Autodesk Fusion 360 part; units mm, degrees
(part 4 of 5)
equation "d217 = SlotWidth"
equation "d218 = ( Depth ) - 2 * ( Wall + DeckClearance + RimBorder )"
equation "d219 = DeckThick"
equation "d221 = TouchChamfer"
equation "d222 = FootHeight"
equation "d224 = ( BaseX ) + ( 0 mm )"
equation "d225 = ( BaseY ) + ( 0 mm )"
equation "d226 = TowerWidth"
equation "d227 = Depth"
equation "d228 = PanHeight + RimLift"
equation "d232 = ( BaseX ) + ( Wall )"
equation "d234 = -( -( ( FootHeight ) + FloorMin + ( ( Depth ) - ( Wall ) ) * tan(DrainSlope) ) )"
equation "d235 = ( ( BaseY ) + ( Wall ) )"
equation "d236 = -( -( ( FootHeight ) + FloorMin + ( ( Depth ) - ( Depth ) ) * tan(DrainSlope) ) )"
equation "d237 = ( ( BaseY ) + ( Depth ) )"
equation "d238 = -( -( FootHeight + PanHeight + RimLift + 1 mm ) )"
equation "d239 = ( TowerWidth ) - 2 * Wall"
equation "d241 = FootHeight"
equation "d243 = ( ( BaseX ) + ( Wall ) )"
equation "d244 = ( ( BaseY ) + ( Wall ) )"
equation "d245 = ( ( BaseX ) + ( Wall + SeatReach ) )"
equation "d246 = ( ( BaseY ) + ( ( Wall ) + SeatLength / 2 ) )"
equation "d247 = ( ( BaseY ) + ( ( Wall ) + SeatLength ) )"
equation "d248 = PanHeight - DeckThick"
equation "d251 = SeatTipRadius"
equation "d252 = FootHeight"
equation "d254 = ( ( BaseX ) + ( Wall ) )"
equation "d255 = ( ( BaseY ) + ( ( Depth ) - Wall - SeatLength ) )"
equation "d256 = ( ( BaseX ) + ( Wall + SeatReach ) )"
equation "d257 = ( ( BaseY ) + ( ( ( Depth ) - Wall - SeatLength ) + SeatLength / 2 ) )"
equation "d258 = ( ( BaseY ) + ( ( ( Depth ) - Wall - SeatLength ) + SeatLength ) )"
equation "d259 = PanHeight - DeckThick"
equation "d262 = SeatTipRadius"
equation "d263 = FootHeight"
equation "d265 = ( ( BaseX ) + ( ( TowerWidth ) - Wall ) )"
equation "d266 = ( ( BaseY ) + ( Wall ) )"
equation "d267 = ( ( BaseX ) + ( ( TowerWidth ) - Wall - SeatReach ) )"
equation "d268 = ( ( BaseY ) + ( ( Wall ) + SeatLength / 2 ) )"
equation "d269 = ( ( BaseY ) + ( ( Wall ) + SeatLength ) )"
equation "d270 = PanHeight - DeckThick"
equation "d273 = SeatTipRadius"
equation "d274 = FootHeight"
equation "d276 = ( ( BaseX ) + ( ( TowerWidth ) - Wall ) )"
equation "d277 = ( ( BaseY ) + ( ( Depth ) - Wall - SeatLength ) )"
equation "d278 = ( ( BaseX ) + ( ( TowerWidth ) - Wall - SeatReach ) )"
equation "d279 = ( ( BaseY ) + ( ( ( Depth ) - Wall - SeatLength ) + SeatLength / 2 ) )"
equation "d280 = ( ( BaseY ) + ( ( ( Depth ) - Wall - SeatLength ) + SeatLength ) )"
equation "d281 = PanHeight - DeckThick"
equation "d284 = SeatTipRadius"
equation "d287 = ( BaseX ) + ( 3 mm )"
equation "d288 = ( BaseY ) + ( 0 mm )"
equation "d289 = RunnerWidth"
equation "d290 = ( Depth ) - 9 mm"
equation "d291 = FootHeight"
equation "d295 = ( BaseX ) + ( ( TowerWidth ) - 3 mm - RunnerWidth )"
equation "d296 = ( BaseY ) + ( 0 mm )"
equation "d297 = RunnerWidth"
equation "d298 = ( Depth ) - 9 mm"
equation "d299 = FootHeight"
equation "d301 = TouchChamfer"
equation "d302 = ( FootHeight ) + PanHeight - DeckThick"
equation "d304 = ( BaseX ) + ( Wall + DeckClearance )"
equation "d305 = ( BaseY ) + ( Wall + DeckClearance )"
equation "d306 = ( TowerWidth ) - 2 * ( Wall + DeckClearance )"
equation "d307 = ( Depth ) - 2 * ( Wall + DeckClearance )"
equation "d308 = DeckThick"
equation "d310 = ( FootHeight ) + PanHeight - DeckThick"
equation "d312 = ( BaseX ) + ( ( ( ( TowerWidth ) - ( 14 * SlotPitch + SlotWidth ) ) / 2 ) + ( 0 * SlotPitch ) )"
equation "d313 = ( BaseY ) + ( Wall + DeckClearance + RimBorder )"
equation "d314 = SlotWidth"
equation "d315 = ( Depth ) - 2 * ( Wall + DeckClearance + RimBorder )"
equation "d316 = DeckThick"
equation "d318 = ( FootHeight ) + PanHeight - DeckThick"
equation "d320 = ( BaseX ) + ( ( ( ( TowerWidth ) - ( 14 * SlotPitch + SlotWidth ) ) / 2 ) + ( 1 * SlotPitch ) )"
equation "d321 = ( BaseY ) + ( Wall + DeckClearance + RimBorder )"
equation "d322 = SlotWidth"
equation "d323 = ( Depth ) - 2 * ( Wall + DeckClearance + RimBorder )"
equation "d324 = DeckThick"
equation "d326 = ( FootHeight ) + PanHeight - DeckThick"
equation "d328 = ( BaseX ) + ( ( ( ( TowerWidth ) - ( 14 * SlotPitch + SlotWidth ) ) / 2 ) + ( 2 * SlotPitch ) )"
equation "d329 = ( BaseY ) + ( Wall + DeckClearance + RimBorder )"
equation "d330 = SlotWidth"
equation "d331 = ( Depth ) - 2 * ( Wall + DeckClearance + RimBorder )"
equation "d332 = DeckThick"
equation "d334 = ( FootHeight ) + PanHeight - DeckThick"
equation "d336 = ( BaseX ) + ( ( ( ( TowerWidth ) - ( 14 * SlotPitch + SlotWidth ) ) / 2 ) + ( 3 * SlotPitch ) )"
equation "d337 = ( BaseY ) + ( Wall + DeckClearance + RimBorder )"
equation "d338 = SlotWidth"
equation "d339 = ( Depth ) - 2 * ( Wall + DeckClearance + RimBorder )"
equation "d340 = DeckThick"
equation "d342 = ( FootHeight ) + PanHeight - DeckThick"
equation "d344 = ( BaseX ) + ( ( ( ( TowerWidth ) - ( 14 * SlotPitch + SlotWidth ) ) / 2 ) + ( 4 * SlotPitch ) )"
equation "d345 = ( BaseY ) + ( Wall + DeckClearance + RimBorder )"
equation "d346 = SlotWidth"
equation "d347 = ( Depth ) - 2 * ( Wall + DeckClearance + RimBorder )"
equation "d348 = DeckThick"
equation "d350 = ( FootHeight ) + PanHeight - DeckThick"
equation "d352 = ( BaseX ) + ( ( ( ( TowerWidth ) - ( 14 * SlotPitch + SlotWidth ) ) / 2 ) + ( 5 * SlotPitch ) )"
equation "d353 = ( BaseY ) + ( Wall + DeckClearance + RimBorder )"
equation "d354 = SlotWidth"
equation "d355 = ( Depth ) - 2 * ( Wall + DeckClearance + RimBorder )"
equation "d356 = DeckThick"
equation "d358 = ( FootHeight ) + PanHeight - DeckThick"
equation "d360 = ( BaseX ) + ( ( ( ( TowerWidth ) - ( 14 * SlotPitch + SlotWidth ) ) / 2 ) + ( 6 * SlotPitch ) )"
equation "d361 = ( BaseY ) + ( Wall + DeckClearance + RimBorder )"
equation "d362 = SlotWidth"
equation "d363 = ( Depth ) - 2 * ( Wall + DeckClearance + RimBorder )"
equation "d364 = DeckThick"
equation "d366 = ( FootHeight ) + PanHeight - DeckThick"
equation "d368 = ( BaseX ) + ( ( ( ( TowerWidth ) - ( 14 * SlotPitch + SlotWidth ) ) / 2 ) + ( 7 * SlotPitch ) )"
equation "d369 = ( BaseY ) + ( Wall + DeckClearance + RimBorder )"
equation "d370 = SlotWidth"
equation "d371 = ( Depth ) - 2 * ( Wall + DeckClearance + RimBorder )"
equation "d372 = DeckThick"
equation "d374 = ( FootHeight ) + PanHeight - DeckThick"
equation "d376 = ( BaseX ) + ( ( ( ( TowerWidth ) - ( 14 * SlotPitch + SlotWidth ) ) / 2 ) + ( 8 * SlotPitch ) )"
equation "d377 = ( BaseY ) + ( Wall + DeckClearance + RimBorder )"
equation "d378 = SlotWidth"
equation "d379 = ( Depth ) - 2 * ( Wall + DeckClearance + RimBorder )"
equation "d380 = DeckThick"
equation "d382 = ( FootHeight ) + PanHeight - DeckThick"
equation "d384 = ( BaseX ) + ( ( ( ( TowerWidth ) - ( 14 * SlotPitch + SlotWidth ) ) / 2 ) + ( 9 * SlotPitch ) )"
equation "d385 = ( BaseY ) + ( Wall + DeckClearance + RimBorder )"
equation "d386 = SlotWidth"
equation "d387 = ( Depth ) - 2 * ( Wall + DeckClearance + RimBorder )"
equation "d388 = DeckThick"
equation "d390 = ( FootHeight ) + PanHeight - DeckThick"
equation "d392 = ( BaseX ) + ( ( ( ( TowerWidth ) - ( 14 * SlotPitch + SlotWidth ) ) / 2 ) + ( 10 * SlotPitch ) )"
equation "d393 = ( BaseY ) + ( Wall + DeckClearance + RimBorder )"
equation "d394 = SlotWidth"
equation "d395 = ( Depth ) - 2 * ( Wall + DeckClearance + RimBorder )"
equation "d396 = DeckThick"
equation "d398 = ( FootHeight ) + PanHeight - DeckThick"
equation "d400 = ( BaseX ) + ( ( ( ( TowerWidth ) - ( 14 * SlotPitch + SlotWidth ) ) / 2 ) + ( 11 * SlotPitch ) )"
equation "d401 = ( BaseY ) + ( Wall + DeckClearance + RimBorder )"
equation "d402 = SlotWidth"
equation "d403 = ( Depth ) - 2 * ( Wall + DeckClearance + RimBorder )"
equation "d404 = DeckThick"
equation "d406 = ( FootHeight ) + PanHeight - DeckThick"
equation "d408 = ( BaseX ) + ( ( ( ( TowerWidth ) - ( 14 * SlotPitch + SlotWidth ) ) / 2 ) + ( 12 * SlotPitch ) )"
equation "d409 = ( BaseY ) + ( Wall + DeckClearance + RimBorder )"
equation "d410 = SlotWidth"
equation "d411 = ( Depth ) - 2 * ( Wall + DeckClearance + RimBorder )"
equation "d412 = DeckThick"
equation "d414 = ( FootHeight ) + PanHeight - DeckThick"
equation "d416 = ( BaseX ) + ( ( ( ( TowerWidth ) - ( 14 * SlotPitch + SlotWidth ) ) / 2 ) + ( 13 * SlotPitch ) )"
equation "d417 = ( BaseY ) + ( Wall + DeckClearance + RimBorder )"
equation "d418 = SlotWidth"
equation "d419 = ( Depth ) - 2 * ( Wall + DeckClearance + RimBorder )"
equation "d420 = DeckThick"
equation "d422 = ( FootHeight ) + PanHeight - DeckThick"
equation "d424 = ( BaseX ) + ( ( ( ( TowerWidth ) - ( 14 * SlotPitch + SlotWidth ) ) / 2 ) + ( 14 * SlotPitch ) )"
equation "d425 = ( BaseY ) + ( Wall + DeckClearance + RimBorder )"
equation "d426 = SlotWidth"
equation "d427 = ( Depth ) - 2 * ( Wall + DeckClearance + RimBorder )"
equation "d428 = DeckThick"
equation "d430 = TouchChamfer"
equation "d431 = FootHeight"
equation "d433 = ( BaseX + TowerWidth + ModuleGap ) + ( 0 mm )"
equation "d434 = ( BaseY ) + ( 0 mm )"
equation "d435 = LeftRun - TowerWidth - ModuleGap"
equation "d436 = Depth"
equation "d437 = PanHeight + RimLift"
equation "d441 = ( BaseX + TowerWidth + ModuleGap ) + ( Wall )"
equation "d443 = -( -( ( FootHeight ) + FloorMin + ( ( Depth ) - ( Wall ) ) * tan(DrainSlope) ) )"
equation "d444 = ( ( BaseY ) + ( Wall ) )"
equation "d445 = -( -( ( FootHeight ) + FloorMin + ( ( Depth ) - ( Depth ) ) * tan(DrainSlope) ) )"
equation "d446 = ( ( BaseY ) + ( Depth ) )"
equation "d447 = -( -( FootHeight + PanHeight + RimLift + 1 mm ) )"
equation "d448 = ( LeftRun - TowerWidth - ModuleGap ) - 2 * Wall"
equation "d450 = FootHeight"
equation "d452 = ( ( BaseX + TowerWidth + ModuleGap ) + ( Wall ) )"
equation "d453 = ( ( BaseY ) + ( Wall ) )"
equation "d454 = ( ( BaseX + TowerWidth + ModuleGap ) + ( Wall + SeatReach ) )"
equation "d455 = ( ( BaseY ) + ( ( Wall ) + SeatLength / 2 ) )"
equation "d456 = ( ( BaseY ) + ( ( Wall ) + SeatLength ) )"
equation "d457 = PanHeight - DeckThick"
equation "d460 = SeatTipRadius"
equation "d461 = FootHeight"
equation "d463 = ( ( BaseX + TowerWidth + ModuleGap ) + ( Wall ) )"
equation "d464 = ( ( BaseY ) + ( ( Depth ) - Wall - SeatLength ) )"
equation "d465 = ( ( BaseX + TowerWidth + ModuleGap ) + ( Wall + SeatReach ) )"
equation "d466 = ( ( BaseY ) + ( ( ( Depth ) - Wall - SeatLength ) + SeatLength / 2 ) )"
equation "d467 = ( ( BaseY ) + ( ( ( Depth ) - Wall - SeatLength ) + SeatLength ) )"
equation "d468 = PanHeight - DeckThick"
equation "d471 = SeatTipRadius"
equation "d472 = FootHeight"
equation "d474 = ( ( BaseX + TowerWidth + ModuleGap ) + ( ( LeftRun - TowerWidth - ModuleGap ) - Wall ) )"
equation "d475 = ( ( BaseY ) + ( Wall ) )"
equation "d476 = ( ( BaseX + TowerWidth + ModuleGap ) + ( ( LeftRun - TowerWidth - ModuleGap ) - Wall - SeatReach ) )"
equation "d477 = ( ( BaseY ) + ( ( Wall ) + SeatLength / 2 ) )"
equation "d478 = ( ( BaseY ) + ( ( Wall ) + SeatLength ) )"
equation "d479 = PanHeight - DeckThick"
equation "d482 = SeatTipRadius"
equation "d483 = FootHeight"
equation "d485 = ( ( BaseX + TowerWidth + ModuleGap ) + ( ( LeftRun - TowerWidth - ModuleGap ) - Wall ) )"
equation "d486 = ( ( BaseY ) + ( ( Depth ) - Wall - SeatLength ) )"
equation "d487 = ( ( BaseX + TowerWidth + ModuleGap ) + ( ( LeftRun - TowerWidth - ModuleGap ) - Wall - SeatReach ) )"
equation "d488 = ( ( BaseY ) + ( ( ( Depth ) - Wall - SeatLength ) + SeatLength / 2 ) )"
equation "d489 = ( ( BaseY ) + ( ( ( Depth ) - Wall - SeatLength ) + SeatLength ) )"
equation "d490 = PanHeight - DeckThick"
equation "d493 = SeatTipRadius"
equation "d496 = ( BaseX + TowerWidth + ModuleGap ) + ( 3 mm )"
equation "d497 = ( BaseY ) + ( 0 mm )"
equation "d498 = RunnerWidth"
equation "d499 = ( Depth ) - 9 mm"
equation "d500 = FootHeight"
equation "d504 = ( BaseX + TowerWidth + ModuleGap ) + ( ( LeftRun - TowerWidth - ModuleGap ) - 3 mm - RunnerWidth )"
equation "d505 = ( BaseY ) + ( 0 mm )"
equation "d506 = RunnerWidth"
equation "d507 = ( Depth ) - 9 mm"
equation "d508 = FootHeight"
equation "d510 = TouchChamfer"
equation "d511 = ( FootHeight ) + PanHeight - DeckThick"
equation "d513 = ( BaseX + TowerWidth + ModuleGap ) + ( Wall + DeckClearance )"
equation "d514 = ( BaseY ) + ( Wall + DeckClearance )"
equation "d515 = ( LeftRun - TowerWidth - ModuleGap ) - 2 * ( Wall + DeckClearance )"
equation "d516 = ( Depth ) - 2 * ( Wall + DeckClearance )"
equation "d517 = DeckThick"
equation "d519 = ( FootHeight ) + PanHeight - DeckThick"
equation "d521 = ( BaseX + TowerWidth + ModuleGap ) + ( ( ( ( LeftRun - TowerWidth - ModuleGap ) - ( 16 * SlotPitch + SlotWidth ) ) / 2 ) + ( 0 * SlotPitch ) )"
equation "d522 = ( BaseY ) + ( Wall + DeckClearance + RimBorder )"
equation "d523 = SlotWidth"
equation "d524 = ( Depth ) - 2 * ( Wall + DeckClearance + RimBorder )"
equation "d525 = DeckThick"
equation "d527 = ( FootHeight ) + PanHeight - DeckThick"
equation "d529 = ( BaseX + TowerWidth + ModuleGap ) + ( ( ( ( LeftRun - TowerWidth - ModuleGap ) - ( 16 * SlotPitch + SlotWidth ) ) / 2 ) + ( 1 * SlotPitch ) )"
equation "d530 = ( BaseY ) + ( Wall + DeckClearance + RimBorder )"
equation "d531 = SlotWidth"
equation "d532 = ( Depth ) - 2 * ( Wall + DeckClearance + RimBorder )"
equation "d533 = DeckThick"
equation "d535 = ( FootHeight ) + PanHeight - DeckThick"
equation "d537 = ( BaseX + TowerWidth + ModuleGap ) + ( ( ( ( LeftRun - TowerWidth - ModuleGap ) - ( 16 * SlotPitch + SlotWidth ) ) / 2 ) + ( 2 * SlotPitch ) )"
equation "d538 = ( BaseY ) + ( Wall + DeckClearance + RimBorder )"
equation "d539 = SlotWidth"
equation "d540 = ( Depth ) - 2 * ( Wall + DeckClearance + RimBorder )"
equation "d541 = DeckThick"
equation "d543 = ( FootHeight ) + PanHeight - DeckThick"
equation "d545 = ( BaseX + TowerWidth + ModuleGap ) + ( ( ( ( LeftRun - TowerWidth - ModuleGap ) - ( 16 * SlotPitch + SlotWidth ) ) / 2 ) + ( 3 * SlotPitch ) )"
equation "d546 = ( BaseY ) + ( Wall + DeckClearance + RimBorder )"
equation "d547 = SlotWidth"
equation "d548 = ( Depth ) - 2 * ( Wall + DeckClearance + RimBorder )"
equation "d549 = DeckThick"
equation "d551 = ( FootHeight ) + PanHeight - DeckThick"
equation "d553 = ( BaseX + TowerWidth + ModuleGap ) + ( ( ( ( LeftRun - TowerWidth - ModuleGap ) - ( 16 * SlotPitch + SlotWidth ) ) / 2 ) + ( 4 * SlotPitch ) )"
equation "d554 = ( BaseY ) + ( Wall + DeckClearance + RimBorder )"
equation "d555 = SlotWidth"
equation "d556 = ( Depth ) - 2 * ( Wall + DeckClearance + RimBorder )"
equation "d557 = DeckThick"
equation "d559 = ( FootHeight ) + PanHeight - DeckThick"
equation "d561 = ( BaseX + TowerWidth + ModuleGap ) + ( ( ( ( LeftRun - TowerWidth - ModuleGap ) - ( 16 * SlotPitch + SlotWidth ) ) / 2 ) + ( 5 * SlotPitch ) )"
equation "d562 = ( BaseY ) + ( Wall + DeckClearance + RimBorder )"
equation "d563 = SlotWidth"
equation "d564 = ( Depth ) - 2 * ( Wall + DeckClearance + RimBorder )"
equation "d565 = DeckThick"
equation "d567 = ( FootHeight ) + PanHeight - DeckThick"
equation "d569 = ( BaseX + TowerWidth + ModuleGap ) + ( ( ( ( LeftRun - TowerWidth - ModuleGap ) - ( 16 * SlotPitch + SlotWidth ) ) / 2 ) + ( 6 * SlotPitch ) )"
equation "d570 = ( BaseY ) + ( Wall + DeckClearance + RimBorder )"
equation "d571 = SlotWidth"
equation "d572 = ( Depth ) - 2 * ( Wall + DeckClearance + RimBorder )"
equation "d573 = DeckThick"
equation "d575 = ( FootHeight ) + PanHeight - DeckThick"
equation "d577 = ( BaseX + TowerWidth + ModuleGap ) + ( ( ( ( LeftRun - TowerWidth - ModuleGap ) - ( 16 * SlotPitch + SlotWidth ) ) / 2 ) + ( 7 * SlotPitch ) )"
equation "d578 = ( BaseY ) + ( Wall + DeckClearance + RimBorder )"
equation "d579 = SlotWidth"
equation "d580 = ( Depth ) - 2 * ( Wall + DeckClearance + RimBorder )"
equation "d581 = DeckThick"
equation "d583 = ( FootHeight ) + PanHeight - DeckThick"
equation "d585 = ( BaseX + TowerWidth + ModuleGap ) + ( ( ( ( LeftRun - TowerWidth - ModuleGap ) - ( 16 * SlotPitch + SlotWidth ) ) / 2 ) + ( 8 * SlotPitch ) )"
equation "d586 = ( BaseY ) + ( Wall + DeckClearance + RimBorder )"
equation "d587 = SlotWidth"
equation "d588 = ( Depth ) - 2 * ( Wall + DeckClearance + RimBorder )"
equation "d589 = DeckThick"
equation "d591 = ( FootHeight ) + PanHeight - DeckThick"
equation "d593 = ( BaseX + TowerWidth + ModuleGap ) + ( ( ( ( LeftRun - TowerWidth - ModuleGap ) - ( 16 * SlotPitch + SlotWidth ) ) / 2 ) + ( 9 * SlotPitch ) )"
equation "d594 = ( BaseY ) + ( Wall + DeckClearance + RimBorder )"
equation "d595 = SlotWidth"
equation "d596 = ( Depth ) - 2 * ( Wall + DeckClearance + RimBorder )"
equation "d597 = DeckThick"
equation "d599 = ( FootHeight ) + PanHeight - DeckThick"
equation "d601 = ( BaseX + TowerWidth + ModuleGap ) + ( ( ( ( LeftRun - TowerWidth - ModuleGap ) - ( 16 * SlotPitch + SlotWidth ) ) / 2 ) + ( 10 * SlotPitch ) )"
equation "d602 = ( BaseY ) + ( Wall + DeckClearance + RimBorder )"
equation "d603 = SlotWidth"
equation "d604 = ( Depth ) - 2 * ( Wall + DeckClearance + RimBorder )"
equation "d605 = DeckThick"
equation "d607 = ( FootHeight ) + PanHeight - DeckThick"
equation "d609 = ( BaseX + TowerWidth + ModuleGap ) + ( ( ( ( LeftRun - TowerWidth - ModuleGap ) - ( 16 * SlotPitch + SlotWidth ) ) / 2 ) + ( 11 * SlotPitch ) )"
equation "d610 = ( BaseY ) + ( Wall + DeckClearance + RimBorder )"
equation "d611 = SlotWidth"
equation "d612 = ( Depth ) - 2 * ( Wall + DeckClearance + RimBorder )"
equation "d613 = DeckThick"
equation "d615 = ( FootHeight ) + PanHeight - DeckThick"
equation "d617 = ( BaseX + TowerWidth + ModuleGap ) + ( ( ( ( LeftRun - TowerWidth - ModuleGap ) - ( 16 * SlotPitch + SlotWidth ) ) / 2 ) + ( 12 * SlotPitch ) )"
equation "d618 = ( BaseY ) + ( Wall + DeckClearance + RimBorder )"
equation "d619 = SlotWidth"
equation "d620 = ( Depth ) - 2 * ( Wall + DeckClearance + RimBorder )"
equation "d621 = DeckThick"
equation "d623 = ( FootHeight ) + PanHeight - DeckThick"
equation "d625 = ( BaseX + TowerWidth + ModuleGap ) + ( ( ( ( LeftRun - TowerWidth - ModuleGap ) - ( 16 * SlotPitch + SlotWidth ) ) / 2 ) + ( 13 * SlotPitch ) )"
equation "d626 = ( BaseY ) + ( Wall + DeckClearance + RimBorder )"
equation "d627 = SlotWidth"
equation "d628 = ( Depth ) - 2 * ( Wall + DeckClearance + RimBorder )"
equation "d629 = DeckThick"
equation "d631 = ( FootHeight ) + PanHeight - DeckThick"
equation "d633 = ( BaseX + TowerWidth + ModuleGap ) + ( ( ( ( LeftRun - TowerWidth - ModuleGap ) - ( 16 * SlotPitch + SlotWidth ) ) / 2 ) + ( 14 * SlotPitch ) )"
equation "d634 = ( BaseY ) + ( Wall + DeckClearance + RimBorder )"
equation "d635 = SlotWidth"
equation "d636 = ( Depth ) - 2 * ( Wall + DeckClearance + RimBorder )"
equation "d637 = DeckThick"
equation "d639 = ( FootHeight ) + PanHeight - DeckThick"
equation "d641 = ( BaseX + TowerWidth + ModuleGap ) + ( ( ( ( LeftRun - TowerWidth - ModuleGap ) - ( 16 * SlotPitch + SlotWidth ) ) / 2 ) + ( 15 * SlotPitch ) )"
equation "d642 = ( BaseY ) + ( Wall + DeckClearance + RimBorder )"
equation "d643 = SlotWidth"
equation "d644 = ( Depth ) - 2 * ( Wall + DeckClearance + RimBorder )"
equation "d645 = DeckThick"
equation "d647 = ( FootHeight ) + PanHeight - DeckThick"
equation "d649 = ( BaseX + TowerWidth + ModuleGap ) + ( ( ( ( LeftRun - TowerWidth - ModuleGap ) - ( 16 * SlotPitch + SlotWidth ) ) / 2 ) + ( 16 * SlotPitch ) )"
equation "d650 = ( BaseY ) + ( Wall + DeckClearance + RimBorder )"
equation "d651 = SlotWidth"
equation "d652 = ( Depth ) - 2 * ( Wall + DeckClearance + RimBorder )"
equation "d653 = DeckThick"
equation "d655 = TouchChamfer"
equation "d656 = FootHeight"
equation "d658 = ( BaseX + LeftRun + FaucetGap + ( RightRun + ModuleGap ) / 2 ) + ( 0 mm )"
equation "d659 = ( BaseY ) + ( 0 mm )"
equation "d660 = ( RightRun - ModuleGap ) / 2"
equation "d661 = Depth"
equation "d662 = PanHeight + RimLift"
equation "d666 = ( BaseX + LeftRun + FaucetGap + ( RightRun + ModuleGap ) / 2 ) + ( Wall )"
equation "d668 = -( -( ( FootHeight ) + FloorMin + ( ( Depth ) - ( Wall ) ) * tan(DrainSlope) ) )"
equation "d669 = ( ( BaseY ) + ( Wall ) )"
equation "d670 = -( -( ( FootHeight ) + FloorMin + ( ( Depth ) - ( Depth ) ) * tan(DrainSlope) ) )"
equation "d671 = ( ( BaseY ) + ( Depth ) )"
equation "d672 = -( -( FootHeight + PanHeight + RimLift + 1 mm ) )"
equation "d673 = ( ( RightRun - ModuleGap ) / 2 ) - 2 * Wall"
equation "d675 = FootHeight"
equation "d677 = ( ( BaseX + LeftRun + FaucetGap + ( RightRun + ModuleGap ) / 2 ) + ( Wall ) )"
equation "d678 = ( ( BaseY ) + ( Wall ) )"
equation "d679 = ( ( BaseX + LeftRun + FaucetGap + ( RightRun + ModuleGap ) / 2 ) + ( Wall + SeatReach ) )"
equation "d680 = ( ( BaseY ) + ( ( Wall ) + SeatLength / 2 ) )"
equation "d681 = ( ( BaseY ) + ( ( Wall ) + SeatLength ) )"
equation "d682 = PanHeight - DeckThick"
equation "d685 = SeatTipRadius"
equation "d686 = FootHeight"
equation "d688 = ( ( BaseX + LeftRun + FaucetGap + ( RightRun + ModuleGap ) / 2 ) + ( Wall ) )"
equation "d689 = ( ( BaseY ) + ( ( Depth ) - Wall - SeatLength ) )"
equation "d690 = ( ( BaseX + LeftRun + FaucetGap + ( RightRun + ModuleGap ) / 2 ) + ( Wall + SeatReach ) )"
equation "d691 = ( ( BaseY ) + ( ( ( Depth ) - Wall - SeatLength ) + SeatLength / 2 ) )"
equation "d692 = ( ( BaseY ) + ( ( ( Depth ) - Wall - SeatLength ) + SeatLength ) )"
equation "d693 = PanHeight - DeckThick"
equation "d696 = SeatTipRadius"
equation "d697 = FootHeight"
equation "d699 = ( ( BaseX + LeftRun + FaucetGap + ( RightRun + ModuleGap ) / 2 ) + ( ( ( RightRun - ModuleGap ) / 2 ) - Wall ) )"
equation "d700 = ( ( BaseY ) + ( Wall ) )"
equation "d701 = ( ( BaseX + LeftRun + FaucetGap + ( RightRun + ModuleGap ) / 2 ) + ( ( ( RightRun - ModuleGap ) / 2 ) - Wall - SeatReach ) )"
equation "d702 = ( ( BaseY ) + ( ( Wall ) + SeatLength / 2 ) )"
equation "d703 = ( ( BaseY ) + ( ( Wall ) + SeatLength ) )"
equation "d704 = PanHeight - DeckThick"
equation "d707 = SeatTipRadius"
equation "d708 = FootHeight"
equation "d710 = ( ( BaseX + LeftRun + FaucetGap + ( RightRun + ModuleGap ) / 2 ) + ( ( ( RightRun - ModuleGap ) / 2 ) - Wall ) )"
equation "d711 = ( ( BaseY ) + ( ( Depth ) - Wall - SeatLength ) )"
equation "d712 = ( ( BaseX + LeftRun + FaucetGap + ( RightRun + ModuleGap ) / 2 ) + ( ( ( RightRun - ModuleGap ) / 2 ) - Wall - SeatReach ) )"
equation "d713 = ( ( BaseY ) + ( ( ( Depth ) - Wall - SeatLength ) + SeatLength / 2 ) )"
equation "d714 = ( ( BaseY ) + ( ( ( Depth ) - Wall - SeatLength ) + SeatLength ) )"
equation "d715 = PanHeight - DeckThick"
equation "d718 = SeatTipRadius"
equation "d721 = ( BaseX + LeftRun + FaucetGap + ( RightRun + ModuleGap ) / 2 ) + ( 3 mm )"
equation "d722 = ( BaseY ) + ( 0 mm )"
equation "d723 = RunnerWidth"
equation "d724 = ( Depth ) - 9 mm"
equation "d725 = FootHeight"
equation "d729 = ( BaseX + LeftRun + FaucetGap + ( RightRun + ModuleGap ) / 2 ) + ( ( ( RightRun - ModuleGap ) / 2 ) - 3 mm - RunnerWidth )"
equation "d730 = ( BaseY ) + ( 0 mm )"
equation "d731 = RunnerWidth"
equation "d732 = ( Depth ) - 9 mm"
equation "d733 = FootHeight"
equation "d735 = TouchChamfer"
equation "d736 = ( FootHeight ) + PanHeight - DeckThick"
equation "d738 = ( BaseX + LeftRun + FaucetGap + ( RightRun + ModuleGap ) / 2 ) + ( Wall + DeckClearance )"
equation "d739 = ( BaseY ) + ( Wall + DeckClearance )"
equation "d740 = ( ( RightRun - ModuleGap ) / 2 ) - 2 * ( Wall + DeckClearance )"
equation "d741 = ( Depth ) - 2 * ( Wall + DeckClearance )"
equation "d742 = DeckThick"
equation "d744 = ( FootHeight ) + PanHeight - DeckThick"
equation "d746 = ( BaseX + LeftRun + FaucetGap + ( RightRun + ModuleGap ) / 2 ) + ( ( ( ( ( RightRun - ModuleGap ) / 2 ) - ( 10 * SlotPitch + SlotWidth ) ) / 2 ) + ( 0 * SlotPitch ) )"
equation "d747 = ( BaseY ) + ( Wall + DeckClearance + RimBorder )"
equation "d748 = SlotWidth"
equation "d749 = ( Depth ) - 2 * ( Wall + DeckClearance + RimBorder )"
equation "d750 = DeckThick"
equation "d752 = ( FootHeight ) + PanHeight - DeckThick"
equation "d754 = ( BaseX + LeftRun + FaucetGap + ( RightRun + ModuleGap ) / 2 ) + ( ( ( ( ( RightRun - ModuleGap ) / 2 ) - ( 10 * SlotPitch + SlotWidth ) ) / 2 ) + ( 1 * SlotPitch ) )"
equation "d755 = ( BaseY ) + ( Wall + DeckClearance + RimBorder )"
equation "d756 = SlotWidth"
equation "d757 = ( Depth ) - 2 * ( Wall + DeckClearance + RimBorder )"
equation "d758 = DeckThick"
equation "d760 = ( FootHeight ) + PanHeight - DeckThick"
equation "d762 = ( BaseX + LeftRun + FaucetGap + ( RightRun + ModuleGap ) / 2 ) + ( ( ( ( ( RightRun - ModuleGap ) / 2 ) - ( 10 * SlotPitch + SlotWidth ) ) / 2 ) + ( 2 * SlotPitch ) )"
equation "d763 = ( BaseY ) + ( Wall + DeckClearance + RimBorder )"
equation "d764 = SlotWidth"
equation "d765 = ( Depth ) - 2 * ( Wall + DeckClearance + RimBorder )"
equation "d766 = DeckThick"
equation "d768 = ( FootHeight ) + PanHeight - DeckThick"
equation "d770 = ( BaseX + LeftRun + FaucetGap + ( RightRun + ModuleGap ) / 2 ) + ( ( ( ( ( RightRun - ModuleGap ) / 2 ) - ( 10 * SlotPitch + SlotWidth ) ) / 2 ) + ( 3 * SlotPitch ) )"
equation "d771 = ( BaseY ) + ( Wall + DeckClearance + RimBorder )"
equation "d772 = SlotWidth"
equation "d773 = ( Depth ) - 2 * ( Wall + DeckClearance + RimBorder )"
equation "d774 = DeckThick"
equation "d776 = ( FootHeight ) + PanHeight - DeckThick"
equation "d778 = ( BaseX + LeftRun + FaucetGap + ( RightRun + ModuleGap ) / 2 ) + ( ( ( ( ( RightRun - ModuleGap ) / 2 ) - ( 10 * SlotPitch + SlotWidth ) ) / 2 ) + ( 4 * SlotPitch ) )"
equation "d779 = ( BaseY ) + ( Wall + DeckClearance + RimBorder )"
equation "d780 = SlotWidth"
equation "d781 = ( Depth ) - 2 * ( Wall + DeckClearance + RimBorder )"
equation "d782 = DeckThick"
equation "d784 = ( FootHeight ) + PanHeight - DeckThick"
equation "d786 = ( BaseX + LeftRun + FaucetGap + ( RightRun + ModuleGap ) / 2 ) + ( ( ( ( ( RightRun - ModuleGap ) / 2 ) - ( 10 * SlotPitch + SlotWidth ) ) / 2 ) + ( 5 * SlotPitch ) )"
equation "d787 = ( BaseY ) + ( Wall + DeckClearance + RimBorder )"
equation "d788 = SlotWidth"
equation "d789 = ( Depth ) - 2 * ( Wall + DeckClearance + RimBorder )"
equation "d790 = DeckThick"
equation "d792 = ( FootHeight ) + PanHeight - DeckThick"
equation "d794 = ( BaseX + LeftRun + FaucetGap + ( RightRun + ModuleGap ) / 2 ) + ( ( ( ( ( RightRun - ModuleGap ) / 2 ) - ( 10 * SlotPitch + SlotWidth ) ) / 2 ) + ( 6 * SlotPitch ) )"
equation "d795 = ( BaseY ) + ( Wall + DeckClearance + RimBorder )"
equation "d796 = SlotWidth"
equation "d797 = ( Depth ) - 2 * ( Wall + DeckClearance + RimBorder )"
equation "d798 = DeckThick"
equation "d800 = ( FootHeight ) + PanHeight - DeckThick"
equation "d802 = ( BaseX + LeftRun + FaucetGap + ( RightRun + ModuleGap ) / 2 ) + ( ( ( ( ( RightRun - ModuleGap ) / 2 ) - ( 10 * SlotPitch + SlotWidth ) ) / 2 ) + ( 7 * SlotPitch ) )"
equation "d803 = ( BaseY ) + ( Wall + DeckClearance + RimBorder )"
equation "d804 = SlotWidth"
equation "d805 = ( Depth ) - 2 * ( Wall + DeckClearance + RimBorder )"
equation "d806 = DeckThick"
equation "d808 = ( FootHeight ) + PanHeight - DeckThick"
equation "d810 = ( BaseX + LeftRun + FaucetGap + ( RightRun + ModuleGap ) / 2 ) + ( ( ( ( ( RightRun - ModuleGap ) / 2 ) - ( 10 * SlotPitch + SlotWidth ) ) / 2 ) + ( 8 * SlotPitch ) )"
equation "d811 = ( BaseY ) + ( Wall + DeckClearance + RimBorder )"
equation "d812 = SlotWidth"
equation "d813 = ( Depth ) - 2 * ( Wall + DeckClearance + RimBorder )"
equation "d814 = DeckThick"
equation "d816 = ( FootHeight ) + PanHeight - DeckThick"
equation "d818 = ( BaseX + LeftRun + FaucetGap + ( RightRun + ModuleGap ) / 2 ) + ( ( ( ( ( RightRun - ModuleGap ) / 2 ) - ( 10 * SlotPitch + SlotWidth ) ) / 2 ) + ( 9 * SlotPitch ) )"
equation "d819 = ( BaseY ) + ( Wall + DeckClearance + RimBorder )"
equation "d820 = SlotWidth"
equation "d821 = ( Depth ) - 2 * ( Wall + DeckClearance + RimBorder )"
equation "d822 = DeckThick"
equation "d824 = ( FootHeight ) + PanHeight - DeckThick"
equation "d826 = ( BaseX + LeftRun + FaucetGap + ( RightRun + ModuleGap ) / 2 ) + ( ( ( ( ( RightRun - ModuleGap ) / 2 ) - ( 10 * SlotPitch + SlotWidth ) ) / 2 ) + ( 10 * SlotPitch ) )"
equation "d827 = ( BaseY ) + ( Wall + DeckClearance + RimBorder )"
equation "d828 = SlotWidth"
equation "d829 = ( Depth ) - 2 * ( Wall + DeckClearance + RimBorder )"
equation "d830 = DeckThick"
equation "d832 = TouchChamfer"
equation "d833 = FootHeight"
equation "d835 = ( BaseX ) + ( 0 mm )"
equation "d836 = ( BaseY + Depth + ModuleGap ) + ( ( LeftReach ) - ( ( 0 mm ) + ( LeftReach ) ) )"
equation "d837 = LeftSideDepth"
equation "d838 = LeftReach"
equation "d839 = PanHeight + RimLift"
equation "d843 = ( BaseY + Depth + ModuleGap ) + ( ( LeftReach ) - ( Wall ) )"
equation "d845 = ( ( BaseX ) + ( Wall ) )"
equation "d846 = -( -( ( FootHeight ) + FloorMin + ( ( LeftSideDepth ) - ( Wall ) ) * tan(DrainSlope) ) )"
equation "d847 = ( ( BaseX ) + ( LeftSideDepth ) )"
equation "d848 = -( -( ( FootHeight ) + FloorMin + ( ( LeftSideDepth ) - ( LeftSideDepth ) ) * tan(DrainSlope) ) )"
equation "d849 = -( -( FootHeight + PanHeight + RimLift + 1 mm ) )"
equation "d850 = -( -( -( ( LeftReach ) - 2 * Wall ) ) )"
equation "d852 = FootHeight"
equation "d854 = ( ( BaseX ) + ( Wall ) )"
equation "d855 = ( ( BaseY + Depth + ModuleGap ) + ( ( LeftReach ) - ( Wall ) ) )"
equation "d856 = ( ( BaseX ) + ( ( Wall ) + SeatLength / 2 ) )"
equation "d857 = ( ( BaseY + Depth + ModuleGap ) + ( ( LeftReach ) - ( Wall + SeatReach ) ) )"
equation "d858 = ( ( BaseX ) + ( ( Wall ) + SeatLength ) )"
equation "d859 = PanHeight - DeckThick"
equation "d862 = SeatTipRadius"
equation "d863 = FootHeight"
equation "d865 = ( ( BaseX ) + ( ( LeftSideDepth ) - Wall - SeatLength ) )"
equation "d866 = ( ( BaseY + Depth + ModuleGap ) + ( ( LeftReach ) - ( Wall ) ) )"
equation "d867 = ( ( BaseX ) + ( ( ( LeftSideDepth ) - Wall - SeatLength ) + SeatLength / 2 ) )"
equation "d868 = ( ( BaseY + Depth + ModuleGap ) + ( ( LeftReach ) - ( Wall + SeatReach ) ) )"
equation "d869 = ( ( BaseX ) + ( ( ( LeftSideDepth ) - Wall - SeatLength ) + SeatLength ) )"
equation "d870 = PanHeight - DeckThick"
equation "d873 = SeatTipRadius"
equation "d874 = FootHeight"
equation "d876 = ( ( BaseX ) + ( Wall ) )"
equation "d877 = ( ( BaseY + Depth + ModuleGap ) + ( ( LeftReach ) - ( ( LeftReach ) - Wall ) ) )"
equation "d878 = ( ( BaseX ) + ( ( Wall ) + SeatLength / 2 ) )"
equation "d879 = ( ( BaseY + Depth + ModuleGap ) + ( ( LeftReach ) - ( ( LeftReach ) - Wall - SeatReach ) ) )"
equation "d880 = ( ( BaseX ) + ( ( Wall ) + SeatLength ) )"
equation "d881 = PanHeight - DeckThick"
equation "d884 = SeatTipRadius"
equation "d885 = FootHeight"
equation "d887 = ( ( BaseX ) + ( ( LeftSideDepth ) - Wall - SeatLength ) )"
equation "d888 = ( ( BaseY + Depth + ModuleGap ) + ( ( LeftReach ) - ( ( LeftReach ) - Wall ) ) )"
equation "d889 = ( ( BaseX ) + ( ( ( LeftSideDepth ) - Wall - SeatLength ) + SeatLength / 2 ) )"
equation "d890 = ( ( BaseY + Depth + ModuleGap ) + ( ( LeftReach ) - ( ( LeftReach ) - Wall - SeatReach ) ) )"
equation "d891 = ( ( BaseX ) + ( ( ( LeftSideDepth ) - Wall - SeatLength ) + SeatLength ) )"
equation "d892 = PanHeight - DeckThick"
equation "d895 = SeatTipRadius"
equation "d898 = ( BaseX ) + ( 0 mm )"
equation "d899 = ( BaseY + Depth + ModuleGap ) + ( ( LeftReach ) - ( ( 3 mm ) + ( RunnerWidth ) ) )"
equation "d900 = ( LeftSideDepth ) - 9 mm"
equation "d901 = RunnerWidth"
equation "d902 = FootHeight"
equation "d906 = ( BaseX ) + ( 0 mm )"
equation "d907 = ( BaseY + Depth + ModuleGap ) + ( ( LeftReach ) - ( ( ( LeftReach ) - 3 mm - RunnerWidth ) + ( RunnerWidth ) ) )"
equation "d908 = ( LeftSideDepth ) - 9 mm"
equation "d909 = RunnerWidth"
equation "d910 = FootHeight"
equation "d912 = TouchChamfer"
equation "d913 = ( FootHeight ) + PanHeight - DeckThick"
equation "d915 = ( BaseX ) + ( Wall + DeckClearance )"
equation "d916 = ( BaseY + Depth + ModuleGap ) + ( ( LeftReach ) - ( ( Wall + DeckClearance ) + ( ( LeftReach ) - 2 * ( Wall + DeckClearance ) ) ) )"
equation "d917 = ( LeftSideDepth ) - 2 * ( Wall + DeckClearance )"
equation "d918 = ( LeftReach ) - 2 * ( Wall + DeckClearance )"
equation "d919 = DeckThick"
equation "d921 = ( FootHeight ) + PanHeight - DeckThick"
equation "d923 = ( BaseX ) + ( Wall + DeckClearance + RimBorder )"
equation "d924 = ( BaseY + Depth + ModuleGap ) + ( ( LeftReach ) - ( ( ( ( ( LeftReach ) - ( 14 * SlotPitch + SlotWidth ) ) / 2 ) + ( 0 * SlotPitch ) ) + ( SlotWidth ) ) )"
equation "d925 = ( LeftSideDepth ) - 2 * ( Wall + DeckClearance + RimBorder )"
equation "d926 = SlotWidth"
equation "d927 = DeckThick"
equation "d929 = ( FootHeight ) + PanHeight - DeckThick"
equation "d931 = ( BaseX ) + ( Wall + DeckClearance + RimBorder )"
equation "d932 = ( BaseY + Depth + ModuleGap ) + ( ( LeftReach ) - ( ( ( ( ( LeftReach ) - ( 14 * SlotPitch + SlotWidth ) ) / 2 ) + ( 1 * SlotPitch ) ) + ( SlotWidth ) ) )"
equation "d933 = ( LeftSideDepth ) - 2 * ( Wall + DeckClearance + RimBorder )"
equation "d934 = SlotWidth"
equation "d935 = DeckThick"
equation "d937 = ( FootHeight ) + PanHeight - DeckThick"
equation "d939 = ( BaseX ) + ( Wall + DeckClearance + RimBorder )"
equation "d940 = ( BaseY + Depth + ModuleGap ) + ( ( LeftReach ) - ( ( ( ( ( LeftReach ) - ( 14 * SlotPitch + SlotWidth ) ) / 2 ) + ( 2 * SlotPitch ) ) + ( SlotWidth ) ) )"
equation "d941 = ( LeftSideDepth ) - 2 * ( Wall + DeckClearance + RimBorder )"
equation "d942 = SlotWidth"
equation "d943 = DeckThick"
equation "d945 = ( FootHeight ) + PanHeight - DeckThick"
equation "d947 = ( BaseX ) + ( Wall + DeckClearance + RimBorder )"
equation "d948 = ( BaseY + Depth + ModuleGap ) + ( ( LeftReach ) - ( ( ( ( ( LeftReach ) - ( 14 * SlotPitch + SlotWidth ) ) / 2 ) + ( 3 * SlotPitch ) ) + ( SlotWidth ) ) )"
equation "d949 = ( LeftSideDepth ) - 2 * ( Wall + DeckClearance + RimBorder )"
equation "d950 = SlotWidth"
equation "d951 = DeckThick"
equation "d953 = ( FootHeight ) + PanHeight - DeckThick"
equation "d955 = ( BaseX ) + ( Wall + DeckClearance + RimBorder )"
equation "d956 = ( BaseY + Depth + ModuleGap ) + ( ( LeftReach ) - ( ( ( ( ( LeftReach ) - ( 14 * SlotPitch + SlotWidth ) ) / 2 ) + ( 4 * SlotPitch ) ) + ( SlotWidth ) ) )"
equation "d957 = ( LeftSideDepth ) - 2 * ( Wall + DeckClearance + RimBorder )"
equation "d958 = SlotWidth"
equation "d959 = DeckThick"
equation "d961 = ( FootHeight ) + PanHeight - DeckThick"
equation "d963 = ( BaseX ) + ( Wall + DeckClearance + RimBorder )"
equation "d964 = ( BaseY + Depth + ModuleGap ) + ( ( LeftReach ) - ( ( ( ( ( LeftReach ) - ( 14 * SlotPitch + SlotWidth ) ) / 2 ) + ( 5 * SlotPitch ) ) + ( SlotWidth ) ) )"
equation "d965 = ( LeftSideDepth ) - 2 * ( Wall + DeckClearance + RimBorder )"
equation "d966 = SlotWidth"
equation "d967 = DeckThick"
equation "d969 = ( FootHeight ) + PanHeight - DeckThick"
equation "d971 = ( BaseX ) + ( Wall + DeckClearance + RimBorder )"
equation "d972 = ( BaseY + Depth + ModuleGap ) + ( ( LeftReach ) - ( ( ( ( ( LeftReach ) - ( 14 * SlotPitch + SlotWidth ) ) / 2 ) + ( 6 * SlotPitch ) ) + ( SlotWidth ) ) )"
equation "d973 = ( LeftSideDepth ) - 2 * ( Wall + DeckClearance + RimBorder )"
equation "d974 = SlotWidth"
equation "d975 = DeckThick"
equation "d977 = ( FootHeight ) + PanHeight - DeckThick"
equation "d979 = ( BaseX ) + ( Wall + DeckClearance + RimBorder )"
equation "d980 = ( BaseY + Depth + ModuleGap ) + ( ( LeftReach ) - ( ( ( ( ( LeftReach ) - ( 14 * SlotPitch + SlotWidth ) ) / 2 ) + ( 7 * SlotPitch ) ) + ( SlotWidth ) ) )"
equation "d981 = ( LeftSideDepth ) - 2 * ( Wall + DeckClearance + RimBorder )"
equation "d982 = SlotWidth"
equation "d983 = DeckThick"
equation "d985 = ( FootHeight ) + PanHeight - DeckThick"
equation "d987 = ( BaseX ) + ( Wall + DeckClearance + RimBorder )"
equation "d988 = ( BaseY + Depth + ModuleGap ) + ( ( LeftReach ) - ( ( ( ( ( LeftReach ) - ( 14 * SlotPitch + SlotWidth ) ) / 2 ) + ( 8 * SlotPitch ) ) + ( SlotWidth ) ) )"
equation "d989 = ( LeftSideDepth ) - 2 * ( Wall + DeckClearance + RimBorder )"
equation "d990 = SlotWidth"
equation "d991 = DeckThick"
equation "d993 = ( FootHeight ) + PanHeight - DeckThick"
equation "d995 = ( BaseX ) + ( Wall + DeckClearance + RimBorder )"
equation "d996 = ( BaseY + Depth + ModuleGap ) + ( ( LeftReach ) - ( ( ( ( ( LeftReach ) - ( 14 * SlotPitch + SlotWidth ) ) / 2 ) + ( 9 * SlotPitch ) ) + ( SlotWidth ) ) )"
equation "d997 = ( LeftSideDepth ) - 2 * ( Wall + DeckClearance + RimBorder )"
equation "d998 = SlotWidth"
equation "d999 = DeckThick"
equation "d1001 = ( FootHeight ) + PanHeight - DeckThick"
equation "d1003 = ( BaseX ) + ( Wall + DeckClearance + RimBorder )"
equation "d1004 = ( BaseY + Depth + ModuleGap ) + ( ( LeftReach ) - ( ( ( ( ( LeftReach ) - ( 14 * SlotPitch + SlotWidth ) ) / 2 ) + ( 10 * SlotPitch ) ) + ( SlotWidth ) ) )"
equation "d1005 = ( LeftSideDepth ) - 2 * ( Wall + DeckClearance + RimBorder )"
equation "d1006 = SlotWidth"
equation "d1007 = DeckThick"
equation "d1009 = ( FootHeight ) + PanHeight - DeckThick"
equation "d1011 = ( BaseX ) + ( Wall + DeckClearance + RimBorder )"
equation "d1012 = ( BaseY + Depth + ModuleGap ) + ( ( LeftReach ) - ( ( ( ( ( LeftReach ) - ( 14 * SlotPitch + SlotWidth ) ) / 2 ) + ( 11 * SlotPitch ) ) + ( SlotWidth ) ) )"
equation "d1013 = ( LeftSideDepth ) - 2 * ( Wall + DeckClearance + RimBorder )"
equation "d1014 = SlotWidth"
equation "d1015 = DeckThick"
equation "d1017 = ( FootHeight ) + PanHeight - DeckThick"
equation "d1019 = ( BaseX ) + ( Wall + DeckClearance + RimBorder )"
equation "d1020 = ( BaseY + Depth + ModuleGap ) + ( ( LeftReach ) - ( ( ( ( ( LeftReach ) - ( 14 * SlotPitch + SlotWidth ) ) / 2 ) + ( 12 * SlotPitch ) ) + ( SlotWidth ) ) )"
equation "d1021 = ( LeftSideDepth ) - 2 * ( Wall + DeckClearance + RimBorder )"
equation "d1022 = SlotWidth"
equation "d1023 = DeckThick"
equation "d1025 = ( FootHeight ) + PanHeight - DeckThick"
equation "d1027 = ( BaseX ) + ( Wall + DeckClearance + RimBorder )"
equation "d1028 = ( BaseY + Depth + ModuleGap ) + ( ( LeftReach ) - ( ( ( ( ( LeftReach ) - ( 14 * SlotPitch + SlotWidth ) ) / 2 ) + ( 13 * SlotPitch ) ) + ( SlotWidth ) ) )"
equation "d1029 = ( LeftSideDepth ) - 2 * ( Wall + DeckClearance + RimBorder )"
equation "d1030 = SlotWidth"
equation "d1031 = DeckThick"
equation "d1033 = ( FootHeight ) + PanHeight - DeckThick"
equation "d1035 = ( BaseX ) + ( Wall + DeckClearance + RimBorder )"
equation "d1036 = ( BaseY + Depth + ModuleGap ) + ( ( LeftReach ) - ( ( ( ( ( LeftReach ) - ( 14 * SlotPitch + SlotWidth ) ) / 2 ) + ( 14 * SlotPitch ) ) + ( SlotWidth ) ) )"
equation "d1037 = ( LeftSideDepth ) - 2 * ( Wall + DeckClearance + RimBorder )"
equation "d1038 = SlotWidth"
equation "d1039 = DeckThick"
equation "d1041 = TouchChamfer"
equation "d1042 = FootHeight"
equation "d1044 = ( BaseX + LeftRun + FaucetGap + RightRun - RightSideDepth ) + ( ( RightSideDepth ) - ( ( 0 mm ) + ( RightSideDepth ) ) )"
equation "d1045 = ( BaseY + Depth + ModuleGap ) + ( 0 mm )"
equation "d1046 = RightSideDepth"
equation "d1047 = RightReach"
equation "d1048 = PanHeight + RimLift"
equation "d1052 = ( BaseY + Depth + ModuleGap ) + ( Wall )"
equation "d1054 = ( ( BaseX + LeftRun + FaucetGap + RightRun - RightSideDepth ) + ( ( RightSideDepth ) - ( Wall ) ) )"
equation "d1055 = -( -( ( FootHeight ) + FloorMin + ( ( RightSideDepth ) - ( Wall ) ) * tan(DrainSlope) ) )"
equation "d1056 = ( ( BaseX + LeftRun + FaucetGap + RightRun - RightSideDepth ) + ( ( RightSideDepth ) - ( RightSideDepth ) ) )"
equation "d1057 = -( -( ( FootHeight ) + FloorMin + ( ( RightSideDepth ) - ( RightSideDepth ) ) * tan(DrainSlope) ) )"
equation "d1058 = -( -( FootHeight + PanHeight + RimLift + 1 mm ) )"
equation "d1059 = ( RightReach ) - 2 * Wall"
equation "d1061 = FootHeight"
equation "d1063 = ( ( BaseX + LeftRun + FaucetGap + RightRun - RightSideDepth ) + ( ( RightSideDepth ) - ( Wall ) ) )"
equation "d1064 = ( ( BaseY + Depth + ModuleGap ) + ( Wall ) )"
equation "d1065 = ( ( BaseX + LeftRun + FaucetGap + RightRun - RightSideDepth ) + ( ( RightSideDepth ) - ( ( Wall ) + SeatLength / 2 ) ) )"
equation "d1066 = ( ( BaseY + Depth + ModuleGap ) + ( Wall + SeatReach ) )"
equation "d1067 = ( ( BaseX + LeftRun + FaucetGap + RightRun - RightSideDepth ) + ( ( RightSideDepth ) - ( ( Wall ) + SeatLength ) ) )"
equation "d1068 = PanHeight - DeckThick"
equation "d1071 = SeatTipRadius"
equation "d1072 = FootHeight"
equation "d1074 = ( ( BaseX + LeftRun + FaucetGap + RightRun - RightSideDepth ) + ( ( RightSideDepth ) - ( ( RightSideDepth ) - Wall - SeatLength ) ) )"
equation "d1075 = ( ( BaseY + Depth + ModuleGap ) + ( Wall ) )"
equation "d1076 = ( ( BaseX + LeftRun + FaucetGap + RightRun - RightSideDepth ) + ( ( RightSideDepth ) - ( ( ( RightSideDepth ) - Wall - SeatLength ) + SeatLength / 2 ) ) )"
equation "d1077 = ( ( BaseY + Depth + ModuleGap ) + ( Wall + SeatReach ) )"
equation "d1078 = ( ( BaseX + LeftRun + FaucetGap + RightRun - RightSideDepth ) + ( ( RightSideDepth ) - ( ( ( RightSideDepth ) - Wall - SeatLength ) + SeatLength ) ) )"
equation "d1079 = PanHeight - DeckThick"
equation "d1082 = SeatTipRadius"
equation "d1083 = FootHeight"
equation "d1085 = ( ( BaseX + LeftRun + FaucetGap + RightRun - RightSideDepth ) + ( ( RightSideDepth ) - ( Wall ) ) )"
equation "d1086 = ( ( BaseY + Depth + ModuleGap ) + ( ( RightReach ) - Wall ) )"
equation "d1087 = ( ( BaseX + LeftRun + FaucetGap + RightRun - RightSideDepth ) + ( ( RightSideDepth ) - ( ( Wall ) + SeatLength / 2 ) ) )"
equation "d1088 = ( ( BaseY + Depth + ModuleGap ) + ( ( RightReach ) - Wall - SeatReach ) )"
equation "d1089 = ( ( BaseX + LeftRun + FaucetGap + RightRun - RightSideDepth ) + ( ( RightSideDepth ) - ( ( Wall ) + SeatLength ) ) )"
equation "d1090 = PanHeight - DeckThick"
equation "d1093 = SeatTipRadius"
equation "d1094 = FootHeight"
equation "d1096 = ( ( BaseX + LeftRun + FaucetGap + RightRun - RightSideDepth ) + ( ( RightSideDepth ) - ( ( RightSideDepth ) - Wall - SeatLength ) ) )"
equation "d1097 = ( ( BaseY + Depth + ModuleGap ) + ( ( RightReach ) - Wall ) )"
equation "d1098 = ( ( BaseX + LeftRun + FaucetGap + RightRun - RightSideDepth ) + ( ( RightSideDepth ) - ( ( ( RightSideDepth ) - Wall - SeatLength ) + SeatLength / 2 ) ) )"
equation "d1099 = ( ( BaseY + Depth + ModuleGap ) + ( ( RightReach ) - Wall - SeatReach ) )"
equation "d1100 = ( ( BaseX + LeftRun + FaucetGap + RightRun - RightSideDepth ) + ( ( RightSideDepth ) - ( ( ( RightSideDepth ) - Wall - SeatLength ) + SeatLength ) ) )"
equation "d1101 = PanHeight - DeckThick"
equation "d1104 = SeatTipRadius"
equation "d1107 = ( BaseX + LeftRun + FaucetGap + RightRun - RightSideDepth ) + ( ( RightSideDepth ) - ( ( 0 mm ) + ( ( RightSideDepth ) - 9 mm ) ) )"
equation "d1108 = ( BaseY + Depth + ModuleGap ) + ( 3 mm )"
equation "d1109 = ( RightSideDepth ) - 9 mm"
equation "d1110 = RunnerWidth"
equation "d1111 = FootHeight"
equation "d1115 = ( BaseX + LeftRun + FaucetGap + RightRun - RightSideDepth ) + ( ( RightSideDepth ) - ( ( 0 mm ) + ( ( RightSideDepth ) - 9 mm ) ) )"
equation "d1116 = ( BaseY + Depth + ModuleGap ) + ( ( RightReach ) - 3 mm - RunnerWidth )"
equation "d1117 = ( RightSideDepth ) - 9 mm"
equation "d1118 = RunnerWidth"
equation "d1119 = FootHeight"
equation "d1121 = TouchChamfer"
equation "d1122 = ( FootHeight ) + PanHeight - DeckThick"
equation "d1124 = ( BaseX + LeftRun + FaucetGap + RightRun - RightSideDepth ) + ( ( RightSideDepth ) - ( ( Wall + DeckClearance ) + ( ( RightSideDepth ) - 2 * ( Wall + DeckClearance ) ) ) )"
equation "d1125 = ( BaseY + Depth + ModuleGap ) + ( Wall + DeckClearance )"
equation "d1126 = ( RightSideDepth ) - 2 * ( Wall + DeckClearance )"
equation "d1127 = ( RightReach ) - 2 * ( Wall + DeckClearance )"
equation "d1128 = DeckThick"
equation "d1130 = ( FootHeight ) + PanHeight - DeckThick"
equation "d1132 = ( BaseX + LeftRun + FaucetGap + RightRun - RightSideDepth ) + ( ( RightSideDepth ) - ( ( Wall + DeckClearance + RimBorder ) + ( ( RightSideDepth ) - 2 * ( Wall + DeckClearance + RimBorder ) ) ) )"
equation "d1133 = ( BaseY + Depth + ModuleGap ) + ( ( ( ( RightReach ) - ( 14 * SlotPitch + SlotWidth ) ) / 2 ) + ( 0 * SlotPitch ) )"
equation "d1134 = ( RightSideDepth ) - 2 * ( Wall + DeckClearance + RimBorder )"
equation "d1135 = SlotWidth"
equation "d1136 = DeckThick"
equation "d1138 = ( FootHeight ) + PanHeight - DeckThick"
equation "d1140 = ( BaseX + LeftRun + FaucetGap + RightRun - RightSideDepth ) + ( ( RightSideDepth ) - ( ( Wall + DeckClearance + RimBorder ) + ( ( RightSideDepth ) - 2 * ( Wall + DeckClearance + RimBorder ) ) ) )"
equation "d1141 = ( BaseY + Depth + ModuleGap ) + ( ( ( ( RightReach ) - ( 14 * SlotPitch + SlotWidth ) ) / 2 ) + ( 1 * SlotPitch ) )"
equation "d1142 = ( RightSideDepth ) - 2 * ( Wall + DeckClearance + RimBorder )"
equation "d1143 = SlotWidth"
equation "d1144 = DeckThick"
equation "d1146 = ( FootHeight ) + PanHeight - DeckThick"
equation "d1148 = ( BaseX + LeftRun + FaucetGap + RightRun - RightSideDepth ) + ( ( RightSideDepth ) - ( ( Wall + DeckClearance + RimBorder ) + ( ( RightSideDepth ) - 2 * ( Wall + DeckClearance + RimBorder ) ) ) )"
equation "d1149 = ( BaseY + Depth + ModuleGap ) + ( ( ( ( RightReach ) - ( 14 * SlotPitch + SlotWidth ) ) / 2 ) + ( 2 * SlotPitch ) )"
equation "d1150 = ( RightSideDepth ) - 2 * ( Wall + DeckClearance + RimBorder )"
equation "d1151 = SlotWidth"
equation "d1152 = DeckThick"
equation "d1154 = ( FootHeight ) + PanHeight - DeckThick"
equation "d1156 = ( BaseX + LeftRun + FaucetGap + RightRun - RightSideDepth ) + ( ( RightSideDepth ) - ( ( Wall + DeckClearance + RimBorder ) + ( ( RightSideDepth ) - 2 * ( Wall + DeckClearance + RimBorder ) ) ) )"
equation "d1157 = ( BaseY + Depth + ModuleGap ) + ( ( ( ( RightReach ) - ( 14 * SlotPitch + SlotWidth ) ) / 2 ) + ( 3 * SlotPitch ) )"
equation "d1158 = ( RightSideDepth ) - 2 * ( Wall + DeckClearance + RimBorder )"
equation "d1159 = SlotWidth"
equation "d1160 = DeckThick"
equation "d1162 = ( FootHeight ) + PanHeight - DeckThick"
equation "d1164 = ( BaseX + LeftRun + FaucetGap + RightRun - RightSideDepth ) + ( ( RightSideDepth ) - ( ( Wall + DeckClearance + RimBorder ) + ( ( RightSideDepth ) - 2 * ( Wall + DeckClearance + RimBorder ) ) ) )"
equation "d1165 = ( BaseY + Depth + ModuleGap ) + ( ( ( ( RightReach ) - ( 14 * SlotPitch + SlotWidth ) ) / 2 ) + ( 4 * SlotPitch ) )"
equation "d1166 = ( RightSideDepth ) - 2 * ( Wall + DeckClearance + RimBorder )"
equation "d1167 = SlotWidth"
equation "d1168 = DeckThick"
equation "d1170 = ( FootHeight ) + PanHeight - DeckThick"
equation "d1172 = ( BaseX + LeftRun + FaucetGap + RightRun - RightSideDepth ) + ( ( RightSideDepth ) - ( ( Wall + DeckClearance + RimBorder ) + ( ( RightSideDepth ) - 2 * ( Wall + DeckClearance + RimBorder ) ) ) )"
equation "d1173 = ( BaseY + Depth + ModuleGap ) + ( ( ( ( RightReach ) - ( 14 * SlotPitch + SlotWidth ) ) / 2 ) + ( 5 * SlotPitch ) )"
equation "d1174 = ( RightSideDepth ) - 2 * ( Wall + DeckClearance + RimBorder )"
equation "d1175 = SlotWidth"
equation "d1176 = DeckThick"
equation "d1178 = ( FootHeight ) + PanHeight - DeckThick"
equation "d1180 = ( BaseX + LeftRun + FaucetGap + RightRun - RightSideDepth ) + ( ( RightSideDepth ) - ( ( Wall + DeckClearance + RimBorder ) + ( ( RightSideDepth ) - 2 * ( Wall + DeckClearance + RimBorder ) ) ) )"
equation "d1181 = ( BaseY + Depth + ModuleGap ) + ( ( ( ( RightReach ) - ( 14 * SlotPitch + SlotWidth ) ) / 2 ) + ( 6 * SlotPitch ) )"
equation "d1182 = ( RightSideDepth ) - 2 * ( Wall + DeckClearance + RimBorder )"
equation "d1183 = SlotWidth"
equation "d1184 = DeckThick"
equation "d1186 = ( FootHeight ) + PanHeight - DeckThick"
equation "d1188 = ( BaseX + LeftRun + FaucetGap + RightRun - RightSideDepth ) + ( ( RightSideDepth ) - ( ( Wall + DeckClearance + RimBorder ) + ( ( RightSideDepth ) - 2 * ( Wall + DeckClearance + RimBorder ) ) ) )"
equation "d1189 = ( BaseY + Depth + ModuleGap ) + ( ( ( ( RightReach ) - ( 14 * SlotPitch + SlotWidth ) ) / 2 ) + ( 7 * SlotPitch ) )"
equation "d1190 = ( RightSideDepth ) - 2 * ( Wall + DeckClearance + RimBorder )"
equation "d1191 = SlotWidth"
equation "d1192 = DeckThick"
equation "d1194 = ( FootHeight ) + PanHeight - DeckThick"
equation "d1196 = ( BaseX + LeftRun + FaucetGap + RightRun - RightSideDepth ) + ( ( RightSideDepth ) - ( ( Wall + DeckClearance + RimBorder ) + ( ( RightSideDepth ) - 2 * ( Wall + DeckClearance + RimBorder ) ) ) )"
equation "d1197 = ( BaseY + Depth + ModuleGap ) + ( ( ( ( RightReach ) - ( 14 * SlotPitch + SlotWidth ) ) / 2 ) + ( 8 * SlotPitch ) )"
equation "d1198 = ( RightSideDepth ) - 2 * ( Wall + DeckClearance + RimBorder )"
equation "d1199 = SlotWidth"
equation "d1200 = DeckThick"
equation "d1202 = ( FootHeight ) + PanHeight - DeckThick"
equation "d1204 = ( BaseX + LeftRun + FaucetGap + RightRun - RightSideDepth ) + ( ( RightSideDepth ) - ( ( Wall + DeckClearance + RimBorder ) + ( ( RightSideDepth ) - 2 * ( Wall + DeckClearance + RimBorder ) ) ) )"
equation "d1205 = ( BaseY + Depth + ModuleGap ) + ( ( ( ( RightReach ) - ( 14 * SlotPitch + SlotWidth ) ) / 2 ) + ( 9 * SlotPitch ) )"
equation "d1206 = ( RightSideDepth ) - 2 * ( Wall + DeckClearance + RimBorder )"
equation "d1207 = SlotWidth"
equation "d1208 = DeckThick"
equation "d1210 = ( FootHeight ) + PanHeight - DeckThick"
equation "d1212 = ( BaseX + LeftRun + FaucetGap + RightRun - RightSideDepth ) + ( ( RightSideDepth ) - ( ( Wall + DeckClearance + RimBorder ) + ( ( RightSideDepth ) - 2 * ( Wall + DeckClearance + RimBorder ) ) ) )"
equation "d1213 = ( BaseY + Depth + ModuleGap ) + ( ( ( ( RightReach ) - ( 14 * SlotPitch + SlotWidth ) ) / 2 ) + ( 10 * SlotPitch ) )"
equation "d1214 = ( RightSideDepth ) - 2 * ( Wall + DeckClearance + RimBorder )"
equation "d1215 = SlotWidth"
equation "d1216 = DeckThick"
equation "d1218 = ( FootHeight ) + PanHeight - DeckThick"
equation "d1220 = ( BaseX + LeftRun + FaucetGap + RightRun - RightSideDepth ) + ( ( RightSideDepth ) - ( ( Wall + DeckClearance + RimBorder ) + ( ( RightSideDepth ) - 2 * ( Wall + DeckClearance + RimBorder ) ) ) )"
equation "d1221 = ( BaseY + Depth + ModuleGap ) + ( ( ( ( RightReach ) - ( 14 * SlotPitch + SlotWidth ) ) / 2 ) + ( 11 * SlotPitch ) )"
equation "d1222 = ( RightSideDepth ) - 2 * ( Wall + DeckClearance + RimBorder )"
equation "d1223 = SlotWidth"